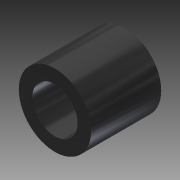
# Autodesk Inventor part: Neoprene Drive Roller 2 in OD 1.94 in Long (2476K33)
Saved by Autodesk Inventor 2014 (Build 180170000, 170)
## iProperties
Created: 2014-01-12
Part Number: Neoprene Drive Roller 2 in OD 1.94 in Long (2476K33)
Material: Rubber
Document SubType Name: Modeling
Designer: Michael
Mass: 56.6005 g
Surface Area: 152.494 cm^2
Volume: 60.8608 cm^3
Density: 0.93 g/cm^3
Appearance: Rubber - Black - Version 1.1
Author: Michael
Autodesk Inventor part; units mm, degrees
ref_plane "YZ Plane" through (0, 0, 0) normal (1, 0, 0) x (0, 1, 0)
ref_plane "XZ Plane" through (0, 0, 0) normal (0, 1, 0) x (-1, 0, 0)
ref_plane "XY Plane" through (0, 0, 0) normal (0, 0, 1) x (1, 0, 0)
sketch "Sketch1" plane through (0, 0, 0) normal (0, 0, 1) x (1, 0, 0)
  circle A0 centre (0, 0) radius 25.4
  circle A1 centre (0, 0) radius 15.875
  dimension "d0" = 50.8
  dimension "d1" = 31.75
  constraints: 2 centre point, 2 coincident
  measures "d0" diameter of A0
  measures "d1" diameter of A1
extrude "Extrusion1" add sketch "Sketch1" along normal blind 49.276
body "Solid1"
